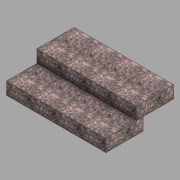
# Autodesk Inventor part: Standard - Steps
Saved by Autodesk Inventor 2022.2 (Build 262287000, 287)
## iProperties
Created: 2022-01-27
Part Number: Standard - Steps
Material: Limestone
Document SubType Name: Modeling
Designer: awelt
Density: 2.6 g/cm^3
Appearance: Mahogany
Author: awelt
Autodesk Inventor part; units mm, degrees
ref_plane "YZ Plane" through (0, 0, 0) normal (1, 0, 0) x (0, 1, 0)
ref_plane "XZ Plane" through (0, 0, 0) normal (0, 1, 0) x (-1, 0, 0)
ref_plane "XY Plane" through (0, 0, 0) normal (0, 0, 1) x (1, 0, 0)
sketch "Sketch1" plane through (0, 0, 0) normal (0, 1, 0) x (-1, 0, 0)
  line L0 (302.0789, 0) -> (-917.1211, 0)
  line L1 (-917.1211, 0) -> (-917.1211, -457.2)
  line L2 (-917.1211, -457.2) -> (302.0789, -457.2)
  line L3 (302.0789, -457.2) -> (302.0789, 0)
  point P0 (0, 0)
  dimension "d0" = 1219.2
  dimension "d1" = 457.2
  constraints: 8 end point, 2 parallel, 1 horizontal, 1 perpendicular
  measures "d0" distance of L2.end L1.end
  measures "d1" distance of L1.end L0.end
extrude "Extrusion1" add sketch "Sketch1" along normal blind 152.4
sketch "Sketch2" plane through (611.9978, 152.4, -833.019) normal (0, 1, 0) x (1, 0, 0)
  line L0 (303.6664, 0) -> (-917.1211, 0)
  line L1 (-917.1211, 0) -> (-917.1211, -457.2)
  line L2 (-917.1211, -457.2) -> (303.6664, -457.2)
  line L3 (303.6664, -457.2) -> (303.6664, 0)
  point P0 (0, 0)
  dimension "d4" = 1220.7875
  dimension "d5" = 457.2
  constraints: 8 end point, 2 parallel, 1 horizontal, 1 perpendicular
  measures "d4" distance of L2.end L1.end
  measures "d5" distance of L1.end L0.end
extrude "Extrusion2" add sketch "Sketch2" along normal blind 152.4 separate body
body "Solid1"
